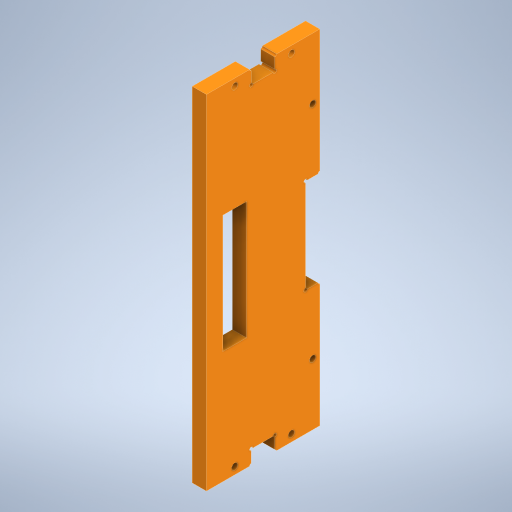
# Autodesk Inventor part: frame_upper4
Saved by Autodesk Inventor 2024 (Build 280153000, 153)
## iProperties
Created: 2024-09-08
Part Number: frame_upper4
Material: 일반
Document SubType Name: Modeling
Designer: jmha0
Density: 1 g/cm^3
Appearance: 주황색
Author: jmha0
Autodesk Inventor part; units mm, degrees
ref_plane "YZ Plane" through (0, 0, 0) normal (1, 0, 0) x (0, 1, 0)
ref_plane "XZ Plane" through (0, 0, 0) normal (0, 1, 0) x (-1, 0, 0)
ref_plane "XY Plane" through (0, 0, 0) normal (0, 0, 1) x (1, 0, 0)
sketch "스케치1" plane through (0, 0, 0) normal (1, 0, 0) x (0, 1, 0)
  circle A0 centre (46.5529, -5.4745) radius 1.35
  circle A1 centre (-46.9471, -5.4745) radius 1.35
  line L0 (-66.9471, -8.4745) -> (66.5529, -8.4745)
  line L1 (66.5529, -8.4745) -> (66.5529, -2.4745)
  line L2 (-66.9471, -2.4745) -> (66.5529, -2.4745)
  line L3 (-66.9471, -8.4745) -> (-66.9471, -2.4745)
  circle A2 centre (-69.9471, 3.5255) radius 1.35
  circle A3 centre (-69.9471, 27.5255) radius 1.35
  line L4 (-66.9471, -8.4745) -> (-66.9471, 39.5255)
  line L5 (-66.9471, 39.5255) -> (-72.9471, 39.5255)
  line L6 (-72.9471, -8.4745) -> (-72.9471, 39.5255)
  line L7 (-66.9471, -8.4745) -> (-72.9471, -8.4745)
  circle A4 centre (69.5529, 3.5255) radius 1.35
  circle A5 centre (69.5529, 27.5255) radius 1.35
  line L8 (72.5529, -8.4745) -> (72.5529, 39.5255)
  line L9 (72.5529, 39.5255) -> (66.5529, 39.5255)
  line L10 (66.5529, -8.4745) -> (66.5529, 39.5255)
  line L11 (72.5529, -8.4745) -> (66.5529, -8.4745)
  point P0 (0, 0)
  constraints: 24 end point, 6 centre point
extrude "돌출1" add sketch "스케치1" along normal blind 6
sketch "스케치3" plane through (0, 66.5529, -2.4745) normal (0, -1, 0) x (1, 0, 0)
  line L0 (0, 42) -> (0, -6) projected
  line L1 (0, 42) -> (0, -6) projected
  line L2 (0, -6) -> (6, -6) projected
  line L3 (6, 42) -> (6, -6) projected
  line L4 (0, 42) -> (6, 42) projected
  line L5 (0, 0) -> (6, 0) projected
  point P0 (0, 2.4745)
  point P1 (0, -6)
extrude "돌출2" add sketch "스케치3" along normal up to surface (133.5 mm away) contours L4 L3 L5 L0
sketch "스케치4" plane through (6, 0, 0) normal (1, 0, 0) x (0, 0, -1)
  line L0 (-39.5255, 72.5529) -> (-39.5255, -72.9471) projected
  line L1 (-39.5255, -72.9471) -> (8.4745, -72.9471) projected
  line L2 (8.4745, -72.9471) -> (8.4745, 72.5529) projected
  line L3 (8.4745, 72.5529) -> (-39.5255, 72.5529) projected
  circle A0 centre (-3.5255, -69.9471) radius 1.35 projected
  circle A1 centre (-27.5255, -69.9471) radius 1.35 projected
  circle A2 centre (5.4745, 46.5529) radius 1.35 projected
  circle A3 centre (5.4745, -46.9471) radius 1.35 projected
  circle A4 centre (-3.5255, 69.5529) radius 1.35 projected
  circle A5 centre (-27.5255, 69.5529) radius 1.35 projected
  line L4 (-20.0255, -25.1971) -> (-35.0255, -25.1971)
  line L5 (-35.0255, -25.1971) -> (-35.0255, 24.8029)
  line L6 (-35.0255, 24.8029) -> (-20.0255, 24.8029)
  line L7 (-20.0255, 24.8029) -> (-20.0255, -25.1971)
  line L8 (-20.0255, -25.1971) -> (-35.0255, 24.8029) construction
  line L9 (-35.0255, -25.1971) -> (-20.0255, 24.8029) construction
  line L10 (-22.5255, -25.1971) -> (-32.5255, -25.1971)
  line L11 (-32.5255, -25.1971) -> (-32.5255, 24.8029)
  line L12 (-32.5255, 24.8029) -> (-22.5255, 24.8029)
  line L13 (-22.5255, 24.8029) -> (-22.5255, -25.1971)
  line L14 (-22.5255, -25.1971) -> (-32.5255, 24.8029) construction
  line L15 (-32.5255, -25.1971) -> (-22.5255, 24.8029) construction
  point P0 (0, 0)
  point P1 (-27.5255, -0.1971)
  dimension "d4" = 15
  dimension "d5" = 50
  dimension "d8" = 10
  dimension "d9" = 50
  constraints: 24 end point, 4 midpoint, 4 parallel, 2 horizontal, 2 perpendicular
  measures "d4" distance of L5.end L6.end
  measures "d5" distance of L4.end L5.end
  measures "d8" distance of L11.end L12.end
  measures "d9" distance of L10.end L11.end
extrude "돌출3" cut sketch "스케치4" against normal blind 10 contours L4 L11 L6 L13
sketch "스케치5" plane through (6, 0, 0) normal (1, 0, 0) x (0, 0, -1)
  line L0 (-32.5255, -25.1971) -> (-32.5255, 24.8029) projected
  line L1 (-32.5255, 24.8029) -> (-22.5255, 24.8029) projected
  line L2 (-22.5255, 24.8029) -> (-22.5255, -25.1971) projected
  line L3 (-22.5255, -25.1971) -> (-32.5255, -25.1971) projected
  line L4 (-39.5255, 72.5529) -> (-39.5255, -72.9471) projected
  line L5 (-39.5255, -72.9471) -> (8.4745, -72.9471) projected
  line L6 (8.4745, -72.9471) -> (8.4745, 72.5529) projected
  line L7 (8.4745, 72.5529) -> (-39.5255, 72.5529) projected
  circle A0 centre (-3.5255, -69.9471) radius 1.35 projected
  circle A1 centre (-27.5255, -69.9471) radius 1.35 projected
  circle A2 centre (5.4745, 46.5529) radius 1.35 projected
  circle A3 centre (5.4745, -46.9471) radius 1.35 projected
  circle A4 centre (-3.5255, 69.5529) radius 1.35 projected
  circle A5 centre (-27.5255, 69.5529) radius 1.35 projected
  line L8 (-10.5255, -72.9471) -> (-20.5255, -72.9471)
  line L9 (-20.5255, -72.9471) -> (-20.5255, -66.9471)
  line L10 (-20.5255, -66.9471) -> (-10.5255, -66.9471)
  line L11 (-10.5255, -66.9471) -> (-10.5255, -72.9471)
  line L12 (-10.5255, -72.9471) -> (-20.5255, -66.9471) construction
  line L13 (-20.5255, -72.9471) -> (-10.5255, -66.9471) construction
  line L14 (-10.5255, 66.5529) -> (-20.5255, 66.5529)
  line L15 (-20.5255, 66.5529) -> (-20.5255, 72.5529)
  line L16 (-20.5255, 72.5529) -> (-10.5255, 72.5529)
  line L17 (-10.5255, 72.5529) -> (-10.5255, 66.5529)
  line L18 (-10.5255, 66.5529) -> (-20.5255, 72.5529) construction
  line L19 (-20.5255, 66.5529) -> (-10.5255, 72.5529) construction
  circle A6 centre (-20.5255, 72.5529) radius 0.75
  circle A7 centre (-20.5255, 66.5529) radius 0.75
  circle A8 centre (-10.5255, 66.5529) radius 0.75
  circle A9 centre (-10.5255, 72.5529) radius 0.75
  circle A10 centre (-20.5255, -66.9471) radius 0.75
  circle A11 centre (-20.5255, -72.9471) radius 0.75
  circle A12 centre (-10.5255, -72.9471) radius 0.75
  circle A13 centre (-10.5255, -66.9471) radius 0.75
  point P0 (0, 0)
  point P1 (-15.5255, -69.9471)
  point P2 (-15.5255, 69.5529)
  point P3 (-20.5255, -72.1971)
  point P4 (-19.7755, -72.9471)
  point P5 (-11.2755, -72.9471)
  point P6 (-10.5255, -72.1971)
  point P7 (-10.5255, -67.6971)
  point P8 (-11.2755, -66.9471)
  point P9 (-19.7755, -66.9471)
  point P10 (-20.5255, -67.6971)
  point P11 (-20.5255, 71.8029)
  point P12 (-20.5255, 67.3029)
  point P13 (-19.7755, 66.5529)
  point P14 (-11.2755, 66.5529)
  point P15 (-10.5255, 67.3029)
  point P16 (-10.5255, 71.8029)
  point P17 (-11.2755, 72.5529)
  point P18 (-19.7755, 72.5529)
  dimension "d10" = 10
  dimension "d11" = 6
  dimension "d12" = 10
  dimension "d13" = 1.5
  dimension "d14" = 1.5
  dimension "d15" = 1.5
  dimension "d16" = 1.5
  dimension "d17" = 1.5
  dimension "d18" = 1.5
  dimension "d19" = 1.5
  dimension "d20" = 1.5
  constraints: 24 end point, 8 centre point, 8 coincident, 4 midpoint, 4 parallel, 2 horizontal, 2 perpendicular, 1 point on line
  measures "d10" distance of L9.end L10.end
  measures "d11" distance of L8.end L9.end
  measures "d12" distance of L15.end L16.end
  measures "d13" diameter of A6
  measures "d14" diameter of A7
  measures "d15" diameter of A8
  measures "d16" diameter of A9
  measures "d17" diameter of A10
  measures "d18" diameter of A11
  measures "d19" diameter of A12
  measures "d20" diameter of A13
extrude "돌출4" cut sketch "스케치5" against normal blind 10 contours A6 L7 | L7 L15 A6 | A11 L9 L5 | L5 A11 | L7 A6 L15 | L7 A9 L17 A8 L14 A7 L15 A6 | L9 A11 L5 | L9 A10 L10 A13 L11 A12 L5 A11 | A9 L7 | L7 L17 A9 | A7 L14 L15 | L15 L14 A7 | A10 L10 L9 | L9 L10 A10 | A12 L11 L5 | L5 A12 | L7 A9 L17 | L11 A12 L5 | A8 L14 L17 | L17 L14 A8 | A13 L11 L10 | L10 L11 A13
sketch "스케치6" plane through (6, 0, 0) normal (1, 0, 0) x (0, 0, -1)
  arc A0 (-9.7755, -72.9471) -> (-10.5255, -72.1971) centre (-10.5255, -72.9471) ccw projected
  line L0 (-9.7755, -72.9471) -> (8.4745, -72.9471) projected
  line L1 (8.4745, -72.9471) -> (8.4745, 72.5529) projected
  line L2 (8.4745, 72.5529) -> (-9.7755, 72.5529) projected
  arc A1 (-10.5255, 71.8029) -> (-9.7755, 72.5529) centre (-10.5255, 72.5529) ccw projected
  line L3 (-10.5255, 71.8029) -> (-10.5255, 67.3029) projected
  arc A2 (-11.2755, 66.5529) -> (-10.5255, 67.3029) centre (-10.5255, 66.5529) ccw projected
  line L4 (-11.2755, 66.5529) -> (-19.7755, 66.5529) projected
  arc A3 (-20.5255, 67.3029) -> (-19.7755, 66.5529) centre (-20.5255, 66.5529) ccw projected
  line L5 (-20.5255, 67.3029) -> (-20.5255, 71.8029) projected
  arc A4 (-21.2755, 72.5529) -> (-20.5255, 71.8029) centre (-20.5255, 72.5529) ccw projected
  line L6 (-21.2755, 72.5529) -> (-39.5255, 72.5529) projected
  line L7 (-39.5255, 72.5529) -> (-39.5255, -72.9471) projected
  line L8 (-39.5255, -72.9471) -> (-21.2755, -72.9471) projected
  arc A5 (-20.5255, -72.1971) -> (-21.2755, -72.9471) centre (-20.5255, -72.9471) ccw projected
  line L9 (-20.5255, -72.1971) -> (-20.5255, -67.6971) projected
  arc A6 (-19.7755, -66.9471) -> (-20.5255, -67.6971) centre (-20.5255, -66.9471) ccw projected
  line L10 (-19.7755, -66.9471) -> (-11.2755, -66.9471) projected
  arc A7 (-10.5255, -67.6971) -> (-11.2755, -66.9471) centre (-10.5255, -66.9471) ccw projected
  line L11 (-10.5255, -67.6971) -> (-10.5255, -72.1971) projected
  line L12 (-32.5255, -25.1971) -> (-32.5255, 24.8029) projected
  line L13 (-32.5255, 24.8029) -> (-22.5255, 24.8029) projected
  line L14 (-22.5255, 24.8029) -> (-22.5255, -25.1971) projected
  line L15 (-22.5255, -25.1971) -> (-32.5255, -25.1971) projected
  circle A8 centre (-3.5255, -69.9471) radius 1.35 projected
  circle A9 centre (-27.5255, -69.9471) radius 1.35 projected
  circle A10 centre (5.4745, 46.5529) radius 1.35 projected
  circle A11 centre (5.4745, -46.9471) radius 1.35 projected
  circle A12 centre (-3.5255, 69.5529) radius 1.35 projected
  circle A13 centre (-27.5255, 69.5529) radius 1.35 projected
  line L16 (8.4745, -72.9471) -> (8.4745, 72.5529) projected
  line L17 (8.4745, -0.1971) -> (5.4745, -0.1971)
  line L18 (2.4745, 19.8029) -> (8.4745, 19.8029)
  line L19 (8.4745, 19.8029) -> (8.4745, -20.1971)
  line L20 (8.4745, -20.1971) -> (2.4745, -20.1971)
  line L21 (2.4745, -20.1971) -> (2.4745, 19.8029)
  line L22 (2.4745, 19.8029) -> (8.4745, -20.1971) construction
  line L23 (8.4745, 19.8029) -> (2.4745, -20.1971) construction
  circle A14 centre (2.4745, -20.1971) radius 0.75
  circle A15 centre (2.4745, 19.8029) radius 0.75
  circle A16 centre (8.4745, 19.8029) radius 0.75
  circle A17 centre (8.4745, -20.1971) radius 0.75
  point P0 (0, 0)
  point P1 (8.4745, 20.5529)
  point P2 (7.7245, 19.8029)
  point P3 (3.2245, 19.8029)
  point P4 (2.4745, 19.0529)
  point P5 (7.7245, -20.1971)
  point P6 (8.4745, -19.4471)
  point P7 (2.4745, -19.4471)
  point P8 (3.2245, -20.1971)
  dimension "d23" = 3
  dimension "d24" = 40
  dimension "d27" = 1.5
  dimension "d28" = 1.5
  dimension "d29" = 1.5
  dimension "d30" = 1.5
  constraints: 14 end point, 4 centre point, 4 coincident, 3 midpoint, 2 horizontal, 2 parallel, 1 perpendicular, 1 point on line
  measures "d23" distance of L17.start L17.end
  measures "d24" distance of L18.end L19.end
  measures "d27" diameter of A14
  measures "d28" diameter of A15
  measures "d29" diameter of A16
  measures "d30" diameter of A17
extrude "돌출5" cut sketch "스케치6" against normal blind 10 contours A17 L20 L1 | L1 A17 | L20 A17 L1 | L20 A14 L21 A15 L18 A16 L1 A17 | A14 L21 L20 | L20 L21 A14 | A16 L18 L1 | A15 L18 L21 | L21 L18 A15 | L18 A16 L1
